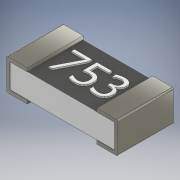
# Autodesk Inventor part: 21-1001
Saved by Autodesk Inventor 2018 (Build 220112000, 112)
## iProperties
Created: 2019-09-21
Part Number: 21-1001
Material: Copper
Document SubType Name: Modeling
Designer: Bradley
Density: 8.94 g/cm^3
Appearance: Smooth - White
Author: Bradley
Autodesk Inventor part; units mm, degrees
ref_plane "YZ Plane" through (0, 0, 0) normal (1, 0, 0) x (0, 1, 0)
ref_plane "XZ Plane" through (0, 0, 0) normal (0, 1, 0) x (-1, 0, 0)
ref_plane "XY Plane" through (0, 0, 0) normal (0, 0, 1) x (1, 0, 0)
sketch "Sketch1" plane through (0, 0, 0) normal (0, 1, 0) x (-1, 0, 0)
  line L0 (0.75, 0.175) -> (-0.75, 0.175)
  line L1 (-0.75, 0.175) -> (-0.75, -0.175)
  line L2 (-0.75, -0.175) -> (0.75, -0.175)
  line L3 (0.75, -0.175) -> (0.75, 0.175)
  line L4 (0.5, 0.175) -> (0.5, 0.225)
  line L5 (0.5, 0.225) -> (0.8, 0.225)
  line L6 (0.8, 0.225) -> (0.8, -0.225)
  line L7 (0.8, -0.225) -> (0.5, -0.225)
  line L8 (0.5, -0.225) -> (0.5, -0.175)
  line L9 (-0.5, 0.175) -> (-0.5, 0.225)
  line L10 (-0.5, 0.225) -> (-0.8, 0.225)
  line L11 (-0.8, 0.225) -> (-0.8, -0.225)
  line L12 (-0.8, -0.225) -> (-0.5, -0.225)
  line L13 (-0.5, -0.175) -> (-0.5, -0.225)
  line L14 (0.5, 0.175) -> (-0.5, 0.175)
  point P0 (0, 0)
  point P1 (0, 0.175)
  point P2 (0.75, 0)
  dimension "d0" = 1.6
  dimension "d1" = 0.05
  dimension "d2" = 0.05
  dimension "d3" = 0.45
  dimension "d4" = 0.3
  constraints: 30 end point, 12 point on line, 7 perpendicular, 3 collinear, 3 midpoint, 2 parallel, 1 horizontal, 1 horizontal alignment, 1 vertical, 1 vertical alignment
  measures "d0" distance between parallel lines of L11 L6
  measures "d1" distance of L7.end L8.end
  measures "d2" distance between parallel lines of L6 L3
  measures "d3" distance of L5.end L6.end
  measures "d4" distance of L6.end L7.end
extrude "Extrusion1" add sketch "Sketch1" along normal mid plane 0.8 contours L0 L4 L5 L6 L7 L8 L2 L3 | L0 L1 L2 L13 L12 L11 L10 L9
extrude "Extrusion2" add sketch "Sketch1" along normal mid plane 0.79 contours L3 L2 L1 L0
sketch "Sketch2" plane through (-0.5, -0.395, 0.175) normal (0, 0, 1) x (1, 0, 0)
  line L0 (0, 0) -> (0, 0.79) projected
  line L1 (1, 0) -> (0, 0) projected
  line L2 (1, 0) -> (1, 0.79) projected
  line L3 (0, 0.79) -> (1, 0.79) projected
  line L4 (0, 0.395) -> (1, 0.395) construction
  line L5 (0.3301, 0.535) -> (0.1571, 0.195)
  line L6 (0.1571, 0.195) -> (0.1, 0.195)
  line L7 (0.1, 0.195) -> (0.2828, 0.548)
  line L8 (0.2828, 0.548) -> (0.0763, 0.548)
  line L9 (0.0763, 0.548) -> (0.0763, 0.595)
  line L10 (0.0763, 0.595) -> (0.3301, 0.595)
  line L11 (0.3301, 0.595) -> (0.3301, 0.535)
  spline S0 degree 2 poles (0.6216, 0.3221) (0.6216, 0.2932) (0.6031, 0.2439) (0.5862, 0.2258) knots 0 0 0 1 2 2 2
  spline S1 degree 2 poles (0.5862, 0.2258) (0.5694, 0.2076) (0.5191, 0.1866) (0.488, 0.1866) knots 0 0 0 1 2 2 2
  spline S2 degree 2 poles (0.488, 0.1866) (0.4595, 0.1866) (0.4037, 0.1992) (0.3833, 0.2093) knots 0 0 0 1 2 2 2
  line L12 (0.3833, 0.2093) -> (0.3833, 0.266)
  line L13 (0.3833, 0.266) -> (0.3872, 0.266)
  spline S3 degree 2 poles (0.3872, 0.266) (0.3934, 0.2615) (0.4164, 0.2498) (0.4303, 0.2446) knots 0 0 0 1 2 2 2
  spline S4 degree 2 poles (0.4303, 0.2446) (0.4462, 0.2391) (0.4724, 0.2329) (0.489, 0.2329) knots 0 0 0 1 2 2 2
  spline S5 degree 2 poles (0.489, 0.2329) (0.5052, 0.2329) (0.5357, 0.2446) (0.5467, 0.2572) knots 0 0 0 1 2 2 2
  spline S6 degree 2 poles (0.5467, 0.2572) (0.5567, 0.2692) (0.5671, 0.301) (0.5671, 0.3224) knots 0 0 0 1 2 2 2
  spline S7 degree 2 poles (0.5671, 0.3224) (0.5671, 0.3438) (0.5554, 0.371) (0.5444, 0.3801) knots 0 0 0 1 2 2 2
  spline S8 degree 2 poles (0.5444, 0.3801) (0.5331, 0.3901) (0.4994, 0.3986) (0.4789, 0.3986) knots 0 0 0 1 2 2 2
  spline S9 degree 2 poles (0.4789, 0.3986) (0.4569, 0.3986) (0.4131, 0.3918) (0.3998, 0.3888) knots 0 0 0 1 2 2 2
  line L14 (0.3998, 0.3888) -> (0.3998, 0.595)
  line L15 (0.3998, 0.595) -> (0.6193, 0.595)
  line L16 (0.6193, 0.595) -> (0.6193, 0.548)
  line L17 (0.6193, 0.548) -> (0.4514, 0.548)
  line L18 (0.4514, 0.548) -> (0.4514, 0.4414)
  spline S10 degree 2 poles (0.4514, 0.4414) (0.4611, 0.4426) (0.4799, 0.4436) (0.4877, 0.4436) knots 0 0 0 1 2 2 2
  spline S11 degree 2 poles (0.4877, 0.4436) (0.5185, 0.4436) (0.5609, 0.4336) (0.5804, 0.4187) knots 0 0 0 1 2 2 2
  spline S12 degree 2 poles (0.5804, 0.4187) (0.6002, 0.4038) (0.6216, 0.3584) (0.6216, 0.3221) knots 0 0 0 1 2 2 2
  spline S13 degree 2 poles (0.7872, 0.5571) (0.7726, 0.5571) (0.7438, 0.5499) (0.7298, 0.5444) knots 0 0 0 1 2 2 2
  spline S14 degree 2 poles (0.7298, 0.5444) (0.7169, 0.5389) (0.6977, 0.5273) (0.6903, 0.5221) knots 0 0 0 1 2 2 2
  line L19 (0.6903, 0.5221) -> (0.687, 0.5221)
  line L20 (0.687, 0.5221) -> (0.687, 0.5788)
  spline S15 degree 2 poles (0.687, 0.5788) (0.7045, 0.5882) (0.7645, 0.6034) (0.7914, 0.6034) knots 0 0 0 1 2 2 2
  spline S16 degree 2 poles (0.7914, 0.6034) (0.8186, 0.6034) (0.8592, 0.5924) (0.8757, 0.5807) knots 0 0 0 1 2 2 2
  spline S17 degree 2 poles (0.8757, 0.5807) (0.8932, 0.5681) (0.9113, 0.5315) (0.9113, 0.5068) knots 0 0 0 1 2 2 2
  spline S18 degree 2 poles (0.9113, 0.5068) (0.9113, 0.4738) (0.8679, 0.4238) (0.8374, 0.4174) knots 0 0 0 1 2 2 2
  line L21 (0.8374, 0.4174) -> (0.8374, 0.4135)
  spline S19 degree 2 poles (0.8374, 0.4135) (0.8501, 0.4109) (0.8789, 0.3992) (0.8912, 0.3875) knots 0 0 0 1 2 2 2
  spline S20 degree 2 poles (0.8912, 0.3875) (0.9036, 0.3762) (0.9191, 0.3399) (0.9191, 0.3136) knots 0 0 0 1 2 2 2
  spline S21 degree 2 poles (0.9191, 0.3136) (0.9191, 0.2867) (0.9006, 0.241) (0.8838, 0.2235) knots 0 0 0 1 2 2 2
  spline S22 degree 2 poles (0.8838, 0.2235) (0.8663, 0.2054) (0.8167, 0.1866) (0.7853, 0.1866) knots 0 0 0 1 2 2 2
  spline S23 degree 2 poles (0.7853, 0.1866) (0.7551, 0.1866) (0.6961, 0.2012) (0.676, 0.2112) knots 0 0 0 1 2 2 2
  line L22 (0.676, 0.2112) -> (0.676, 0.2679)
  line L23 (0.676, 0.2679) -> (0.6799, 0.2679)
  spline S24 degree 2 poles (0.6799, 0.2679) (0.6968, 0.2556) (0.7538, 0.2329) (0.782, 0.2329) knots 0 0 0 1 2 2 2
  spline S25 degree 2 poles (0.782, 0.2329) (0.7985, 0.2329) (0.8316, 0.2433) (0.8426, 0.2553) knots 0 0 0 1 2 2 2
  spline S26 degree 2 poles (0.8426, 0.2553) (0.8533, 0.2673) (0.8647, 0.2958) (0.8647, 0.3175) knots 0 0 0 1 2 2 2
  spline S27 degree 2 poles (0.8647, 0.3175) (0.8647, 0.3392) (0.852, 0.3674) (0.8407, 0.3756) knots 0 0 0 1 2 2 2
  spline S28 degree 2 poles (0.8407, 0.3756) (0.8293, 0.3837) (0.7985, 0.3898) (0.7804, 0.3898) knots 0 0 0 1 2 2 2
  line L24 (0.7804, 0.3898) -> (0.7577, 0.3898)
  line L25 (0.7577, 0.3898) -> (0.7577, 0.4342)
  line L26 (0.7577, 0.4342) -> (0.7755, 0.4342)
  spline S29 degree 2 poles (0.7755, 0.4342) (0.8115, 0.4342) (0.8569, 0.4686) (0.8569, 0.5013) knots 0 0 0 1 2 2 2
  spline S30 degree 2 poles (0.8569, 0.5013) (0.8569, 0.5166) (0.8452, 0.5383) (0.8358, 0.5448) knots 0 0 0 1 2 2 2
  spline S31 degree 2 poles (0.8358, 0.5448) (0.8258, 0.5516) (0.8011, 0.5571) (0.7872, 0.5571) knots 0 0 0 1 2 2 2
  point P0 (0.5, 0.395)
  constraints: 2 end point, 2 midpoint, 1 horizontal
extrude "Extrusion3" add sketch "Sketch2" along normal blind 0.02 contours L5 L6 L7 L8 L9 L10 L11 | S0 S1 S2 L12 L13 S3 S4 S5 S6 S7 S8 S9 L14 L15 L16 L17 L18 S10 S11 S12 | S13 S14 L19 L20 S15 S16 S17 S18 L21 S19 S20 S21 S22 S23 L22 L23 S24 S25 S26 S27 S28 L24 L25 L26 S29 S30 S31
fillet "Fillet1" radius 0.02 4 edges at (-0.8, 0, 0.225) (-0.8, 0, -0.225) (0.8, 0, 0.225) (0.8, 0, -0.225)
equation "\"d2\" = d1"
body "Solid1"
